Autodesk Fusion 360 part; units mm, degrees
(part 2 of 4)
sketch "Esquisse16 (2)" plane through (0, 0, 59.7937) normal (0, 0, 1) x (-1, 0, 0) in component "Left_Bottom_Holder"
  line L0 (-5.3, -152.2) -> (120.3, -152.2)
  line L1 (120.3, -152.2) -> (120.3, -145)
  line L2 (120.3, -145) -> (0, -145)
  line L3 (0, -145) -> (0, 145)
  line L4 (0, 145) -> (120.3, 145)
  line L5 (120.3, 157.8) -> (120.3, 165)
  line L6 (120.3, 165) -> (-20, 165)
  line L7 (-20, 165) -> (-20, -165)
  line L8 (-20, -165) -> (120.3, -165)
  line L9 (120.3, -165) -> (120.3, -157.8)
  line L10 (120.3, -157.8) -> (-5.3, -157.8)
  line L11 (-5.3, -157.8) -> (-5.3, -152.2)
  line L12 (0.0045, -165) -> (120.3, -165) construction
  line L13 (60.1522, -165) -> (60.15, -145) construction
  line L14 (60.1511, -155) -> (47.2609, -155.0014) construction
  line L15 (77.6517, -157.8) -> (42.6517, -157.8)
  line L16 (42.6517, -157.8) -> (42.6517, -160.3)
  line L17 (42.6517, -160.3) -> (77.6517, -160.3)
  line L18 (77.6517, -160.3) -> (77.6517, -157.8)
  line L19 (77.6505, -149.6961) -> (77.6511, -152.1961)
  line L20 (77.6511, -152.1961) -> (42.6511, -152.2039)
  line L21 (0, -145) -> (-20, -145)
  line L22 (-20, -145) -> (-20, -165)
  line L23 (-20, -165) -> (0, -165)
  line L24 (0, -165) -> (0, -145)
  line L25 (-20, 0) -> (0, 0) construction
  line L26 (-12.8, -150.3) -> (-7.2, -150.3)
  line L27 (-7.2, -150.3) -> (-7.2, 150.3)
  line L28 (-7.2, 150.3) -> (-12.8, 150.3)
  line L29 (-12.8, 150.3) -> (-12.8, -150.3)
  line L30 (-10, -165) -> (-10, -145) construction
  line L31 (0, 145) -> (-20, 145)
  line L32 (-20, 145) -> (-20, 165)
  line L33 (-20, 165) -> (0, 165)
  line L34 (0, 165) -> (0, 145)
  line L35 (-12.8, 70) -> (-12.8, -70)
  line L36 (-10, 0) -> (-10, 10) construction
  line L37 (-7.2, 70) -> (-7.2, -70)
  line L38 (0, 165) -> (120.3, 165) construction
  line L39 (60.15, 165) -> (60.15, 145) construction
  line L40 (-5.3, 157.8) -> (120.3, 157.8)
  line L41 (120.3, 152.2) -> (-5.3, 152.2)
  line L42 (-5.3, 152.2) -> (-5.3, 157.8)
  line L43 (-5.3, 157.8) -> (-5.3, 152.2)
  line L44 (-5.3, 152.2) -> (120.3, 152.2)
  line L45 (120.3, 152.2) -> (120.3, 157.8)
  line L46 (120.3, 157.8) -> (-5.3, 157.8)
  line L47 (42.65, 157.8) -> (77.65, 157.8)
  line L48 (77.65, 157.8) -> (77.65, 160.3)
  line L49 (77.65, 160.3) -> (42.65, 160.3)
  line L50 (42.65, 160.3) -> (42.65, 157.8)
  line L51 (60.15, 155) -> (66, 155) construction
  line L52 (42.65, 152.2) -> (77.65, 152.2)
  line L53 (42.65, 149.7) -> (42.65, 152.2)
  line L54 (77.65, 149.7) -> (42.65, 149.7)
  line L55 (77.65, 152.2) -> (77.65, 149.7)
  line L56 (-12.8, -90) -> (-15.3, -90)
  line L57 (-15.3, -90) -> (-15.3, -55)
  line L58 (-15.3, -55) -> (-12.8, -55)
  line L59 (-12.8, -55) -> (-12.8, -90)
  line L60 (-15.3, -90) -> (-15.3, -145) construction
  line L61 (-15.3, -55) -> (-15.3, 0) construction
  line L62 (-4.7, -90) -> (-4.7, -55)
  line L63 (-7.2, -90) -> (-4.7, -90)
  line L64 (-4.7, -55) -> (-7.2, -55)
  line L65 (-7.2, -55) -> (-7.2, -90)
  line L66 (-15.3, 90) -> (-15.3, 55)
  line L67 (-15.3, 55) -> (-12.8, 55)
  line L68 (-4.7, 90) -> (-4.7, 55)
  line L69 (-7.2, 55) -> (-7.2, 90)
  line L70 (-7.2, 90) -> (-4.7, 90)
  line L71 (-4.7, 55) -> (-7.2, 55)
  line L72 (-12.8, 90) -> (-15.3, 90)
  line L73 (-12.8, 55) -> (-12.8, 90)
  line L74 (77.6511, -152.1961) -> (42.6511, -152.2039)
  line L75 (42.6505, -149.7039) -> (77.6505, -149.6961)
  line L76 (42.6511, -152.2039) -> (42.6505, -149.7039)
  line L77 (77.6505, -149.6961) -> (77.6511, -152.1961)
  line L78 (77.6511, -152.1961) -> (42.6511, -152.2039)
  point P0 (60.1517, -160.3)
  point P1 (-10, -150.3)
  point P2 (-12.8, 0)
  point P3 (-15.3, 0)
  point P4 (60.15, 160.3)
  dimension "d128_1" = 2.5
  dimension "d129_1" = 35
  dimension "d145_1" = 5.6
  dimension "d146_1" = 300.6
  dimension "d149_1" = 2.5
  dimension "d150_1" = 35
  dimension "d236" = 2.5
  dimension "d237" = 35
  constraint coincident L8 L12.start
  constraint coincident L8.end L9.start
  constraint midpoint L12 L13.start
  constraint midpoint L2 L13.end
  constraint midpoint L13 L14.start
  constraint perpendicular L13 L14
  constraint horizontal L15
  constraint vertical L16
  constraint horizontal L17
  constraint vertical L18
  constraint coincident L10 L15.start
  constraint midpoint L17 P0
  constraint coincident L13 P0
  constraint symmetric L14 L15.start L19.end
  constraint symmetric L14 L15.end L20.end
  constraint symmetric L14 L17.end L19.start
  constraint horizontal L21
  constraint vertical L22
  constraint horizontal L23
  constraint vertical L24
  constraint coincident L7.end L8.start
  constraint coincident L2.end L3.start
  constraint midpoint L7 L25.start
  constraint coincident L25.end origin
  constraint horizontal L26
  constraint vertical L27
  constraint horizontal L28
  constraint vertical L29
  constraint midpoint L26 P1
  constraint midpoint L23 L30.start
  constraint midpoint L21 L30.end
  constraint coincident P1 L30
  constraint midpoint L29 P2
  constraint coincident L25 P2
  constraint horizontal L31
  constraint vertical L32
  constraint horizontal L33
  constraint vertical L34
  constraint coincident L6.end L7.start
  constraint coincident L3.end L4.start
  constraint vertical L35
  constraint coincident L29 L35.end
  constraint coincident L25 P3
  constraint midpoint L25 L36.start
  constraint perpendicular L25 L36
  constraint symmetric L35.end L36 L37.end
  constraint symmetric L35.start L36 L37.start
  constraint coincident L5.end L6.start
  constraint midpoint L38 L39.start
  constraint midpoint L4 L39.end
  constraint horizontal L47
  constraint vertical L48
  constraint horizontal L49
  constraint vertical L50
  constraint coincident L40 L47.start
  constraint midpoint L49 P4
  constraint coincident L39 P4
  constraint midpoint L39 L51.start
  constraint perpendicular L39 L51
  constraint symmetric L47.start L51 L52.start
  constraint symmetric L47.end L51 L52.end
  constraint symmetric L48.end L51 L54.start
  constraint symmetric L49.end L51 L53.start
  constraint horizontal L56
  constraint vertical L57
  constraint horizontal L58
  constraint vertical L59
  constraint coincident L29 L56.start
  constraint coincident L21 L60.end
  constraint perpendicular L21 L60
  constraint coincident P3 L61.end
  constraint perpendicular L25 L61
  constraint equal L60 L61
  constraint symmetric L36 L56.start L63.start
  constraint symmetric L36 L56.end L62.start
  constraint symmetric L36 L57.end L62.end
  constraint symmetric L36 L58.end L64.end
  constraint symmetric L25 L56.start L72.start
  constraint symmetric L25 L56.end L66.start
  constraint symmetric L25 L57.end L66.end
  constraint symmetric L25 L58.end L67.end
  constraint symmetric L25 L62.start L68.start
  constraint symmetric L25 L62.end L68.end
  constraint symmetric L25 L63.start L69.end
  constraint symmetric L25 L64.end L69.start
  constraint symmetric L14 L16.end L75.start
  measures "d128_1" distance of L15.end L16.end
  measures "d129_1" distance of L16.end L17.end
  measures "d145_1" distance of L26.start L26.end
  measures "d146_1" distance of L26.start L28.end
  measures "d149_1" distance of L47.start L49.end
  measures "d150_1" distance of L48.end L49.end
  measures "d236" distance of L56.start L56.end
  measures "d237" distance of L56.end L57.end
extrude "Extrusion23'" add sketch "Esquisse16 (2)" along normal blind 10 contours L0 L19 L20 L74 L75 L76 L77 L78 | L0 L20 L74 L76 L78 | L10 L15 L16 L17 L18 | L27 L37 L62 L63 L64 L65 | L27 L37 L68 L69 L70 L71 | L41 L44 L52 L53 L54 L55 | L29 L35 L56 L57 L58 L59 | L29 L35 L66 L67 L72 L73 | L40 L46 L47 L48 L49 L50 bodies 4 in component "Left_Bottom_Holder"
extrude "Extrusion28'" cut sketch "Esquisse16 (2)" against normal blind 5.3 contours L21 L26 L27 L29 | L21 L27 L29 L31 L35 L37 L59 L65 L69 L73 | L27 L28 L29 L31 bodies 4 in component "Left_Bottom_Holder"
extrude "Extrusion29'" add sketch "Esquisse16 (2)" along normal blind 30 contours L0 L7 L8 L10 L11 L21 L22 L23 L24 L26 L27 L29 | L6 L7 L27 L28 L29 L31 L32 L33 L34 L40 L41 L42 L43 L44 L46 bodies 4 in component "Left_Bottom_Holder"
sketch "Esquisse19" plane through (0, 0, 89.7937) normal (0, 0, 1) x (-1, 0, 0) in component "Left_Bottom_Holder"
  line L0 (-12.8, -150.3) -> (-12.8, -145)
  line L1 (-12.8, -145) -> (-20, -145)
  line L2 (-20, -145) -> (-20, -165)
  line L3 (-20, -165) -> (0, -165)
  line L4 (0, -165) -> (0, -157.8)
  line L5 (0, -157.8) -> (-5.3, -157.8)
  line L6 (-5.3, -157.8) -> (-5.3, -152.2)
  line L7 (-5.3, -152.2) -> (0, -152.2)
  line L8 (0, -152.2) -> (0, -145)
  line L9 (0, -145) -> (-7.2, -145)
  line L10 (-7.2, -145) -> (-7.2, -150.3)
  line L11 (-7.2, -150.3) -> (-12.8, -150.3)
  line L12 (-20, -155) -> (0, -155) construction
  line L13 (-10, -165) -> (-10, -145) construction
  circle A0 centre (-15, -155) radius 2.5
  line L14 (-10, -165) -> (-20, -165) construction
  line L15 (-15, -165) -> (-15, -145) construction
  line L16 (0, 145) -> (-20, 145) construction
  line L17 (-20, 145) -> (-20, 165) construction
  line L18 (-20, 165) -> (0, 165) construction
  line L19 (0, 165) -> (0, 145) construction
  line L20 (-10, 145) -> (-10, 165) construction
  line L21 (0, 155) -> (-20, 155) construction
  line L22 (-10, 145) -> (-20, 145) construction
  line L23 (-15, 145) -> (-15, 165) construction
  circle A1 centre (-15, 155) radius 2.5
  dimension "d155_1" = 5
  dimension "d375" = 5
  constraint midpoint L2 L12.start
  constraint perpendicular L4 L12
  constraint midpoint L3 L13.start
  constraint perpendicular L1 L13
  constraint coincident L2.end L3.start
  constraint midpoint L14 L15.start
  constraint coincident L1 L15.end
  constraint perpendicular L1 L15
  constraint midpoint A0.centre L15
  constraint horizontal L16
  constraint vertical L17
  constraint horizontal L18
  constraint vertical L19
  constraint midpoint L18 L20.end
  constraint perpendicular L18 L20
  constraint midpoint L17 L21.end
  constraint perpendicular L17 L21
  constraint perpendicular L17 L22
  constraint midpoint L22 L23.start
  constraint coincident L18 L23.end
  constraint perpendicular L18 L23
  constraint midpoint L23 A1.centre
  measures "d155_1" diameter of A0
  measures "d375" diameter of A1
extrude "Extrusion30" add sketch "Esquisse19" along normal blind 10 contours A0 | A1 bodies 4 in component "Left_Bottom_Holder"
split "Scinder1'" by plane through (-120.3, 0, 47.2937) normal (0, 1, 0) bodies 4 makes body 5 at (13.3333, 103.3333, 39.4937) in component "Left_Bottom_Holder"
move_body "Déplacer1'" bodies 4 to x (1, 0, 0) y (0, 1, 0) z (0, 0, 1) at (0, -80, 0) in component "Left_Bottom_Holder"
sketch "Esquisse21 (2)" plane through (0, -80, 0) normal (0, 1, 0) x (-1, 0, 0) in component "Left_Bottom_Holder"
  line L0 (-10, 39.7937) -> (-10, 54.4937) construction
  line L1 (-20, 49.7937) -> (-5, 49.7937) construction
  line L2 (-20, 49.7937) -> (-10, 39.7937) construction
  line L3 (-10, 49.7937) -> (-20, 39.7937) construction
  circle A0 centre (-15, 44.7937) radius 2.65
  line L4 (0, 39.4937) -> (0, 46.8437)
  line L5 (0, 46.8437) -> (-5, 46.8437)
  line L6 (-5, 46.8437) -> (-5, 52.4437)
  line L7 (-5, 52.4437) -> (0, 52.4437)
  line L8 (0, 52.4437) -> (0, 59.7937)
  line L9 (0, 59.7937) -> (-7.2, 59.7937)
  line L10 (-7.2, 59.7937) -> (-7.2, 54.4937)
  line L11 (-7.2, 54.4937) -> (-12.8, 54.4937)
  line L12 (-12.8, 54.4937) -> (-12.8, 59.7937)
  line L13 (-12.8, 59.7937) -> (-20, 59.7937)
  line L14 (-20, 59.7937) -> (-20, 39.4937)
  line L15 (-20, 39.4937) -> (0, 39.4937)
  dimension "d161_1" = 5.3
  constraint coincident L0 L3.start
  constraint coincident L1 L3.start
  constraint midpoint L3 A0.centre
  measures "d161_1" diameter of A0
extrude "Extrusion32'" cut sketch "Esquisse21 (2)" against normal blind 10.3 contours A0 bodies 4 in component "Left_Bottom_Holder"
sketch "Esquisse22 (2)" plane through (0, 0, 0) normal (0, -1, 0) x (1, 0, 0) in component "Left_Bottom_Holder"
  line L0 (10, 39.7937) -> (10, 54.4937) construction
  line L1 (20, 49.7937) -> (5, 49.7937) construction
  line L2 (20, 39.7937) -> (10, 49.7937) construction
  line L3 (10, 39.7937) -> (20, 49.7937) construction
  circle A0 centre (15, 44.7937) radius 2.5
  line L4 (0, 46.8437) -> (0, 39.4937)
  line L5 (0, 39.4937) -> (20, 39.4937)
  line L6 (20, 39.4937) -> (20, 59.7937)
  line L7 (20, 59.7937) -> (12.8, 59.7937)
  line L8 (12.8, 59.7937) -> (12.8, 54.4937)
  line L9 (12.8, 54.4937) -> (7.2, 54.4937)
  line L10 (7.2, 54.4937) -> (7.2, 59.7937)
  line L11 (7.2, 59.7937) -> (0, 59.7937)
  line L12 (0, 59.7937) -> (0, 52.4437)
  line L13 (0, 52.4437) -> (5, 52.4437)
  line L14 (5, 52.4437) -> (5, 46.8437)
  line L15 (5, 46.8437) -> (0, 46.8437)
  dimension "d164_1" = 5
  constraint coincident L1 L2.end
  constraint coincident L0 L2.end
  constraint midpoint L3 A0.centre
  measures "d164_1" diameter of A0
extrude "Extrusion33'" add sketch "Esquisse22 (2)" along normal blind 10 contours A0 bodies 5 in component "Left_Bottom_Holder"
move_body "Déplacer2'" bodies 4 to x (1, 0, 0) y (0, 1, 0) z (0, 0, 1) at (0, 80, 0) in component "Left_Bottom_Holder"
sketch "Esquisse23 (2)" plane through (0, 145, 0) normal (0, -1, 0) x (1, 0, 0) in component "Left_Bottom_Holder"
  line L0 (0, 59.7937) -> (7.2, 59.7937)
  line L1 (7.2, 59.7937) -> (7.2, 89.7937)
  line L2 (7.2, 89.7937) -> (0, 89.7937)
  line L3 (0, 89.7937) -> (0, 59.7937)
  line L4 (12.8, 59.7937) -> (20, 59.7937)
  line L5 (20, 59.7937) -> (20, 89.7937)
  line L6 (20, 89.7937) -> (12.8, 89.7937)
  line L7 (12.8, 89.7937) -> (12.8, 59.7937)
  line L8 (0, 74.7937) -> (7.2, 74.7937) construction
  line L9 (7.2, 74.7937) -> (12.8, 74.7937) construction
  line L10 (10, 74.7937) -> (10, 86.5) construction
  line L11 (7.2, 66.0437) -> (4.7, 66.0437)
  line L12 (4.7, 66.0437) -> (4.7, 83.5437)
  line L13 (4.7, 83.5437) -> (7.2, 83.5437)
  line L14 (7.2, 83.5437) -> (7.2, 66.0437)
  line L15 (15.3, 66.0437) -> (15.3, 83.5437)
  line L16 (15.3, 83.5437) -> (12.8, 83.5437)
  line L17 (12.8, 83.5437) -> (12.8, 66.0437)
  line L18 (12.8, 66.0437) -> (15.3, 66.0437)
  point P0 (4.7, 74.7937)
  dimension "d171_1" = 2.5
  dimension "d172_1" = 17.5
  constraint midpoint L3 L8.start
  constraint midpoint L1 L8.end
  constraint midpoint L7 L9.end
  constraint midpoint L9 L10.start
  constraint perpendicular L9 L10
  constraint horizontal L11
  constraint vertical L12
  constraint horizontal L13
  constraint vertical L14
  constraint coincident L1 L11.start
  constraint midpoint L12 P0
  constraint coincident L8 P0
  constraint symmetric L10 L11.start L17.end
  constraint symmetric L10 L11.end L15.start
  constraint symmetric L10 L12.end L15.end
  constraint symmetric L10 L13.end L16.end
  measures "d171_1" distance of L12.end L13.end
  measures "d172_1" distance of L11.end L12.end
extrude "Extrusion35'" add sketch "Esquisse23 (2)" along normal blind 10 contours L1 L11 L12 L13 L14 | L7 L15 L16 L17 L18 bodies 5 in component "Left_Bottom_Holder"
sketch "Esquisse24 (2)" plane through (0, -145, 0) normal (0, 1, 0) x (-1, 0, 0) in component "Left_Bottom_Holder"
  line L0 (-20, 59.7937) -> (-12.8, 59.7937)
  line L1 (-12.8, 59.7937) -> (-12.8, 89.7937)
  line L2 (-12.8, 89.7937) -> (-20, 89.7937)
  line L3 (-20, 89.7937) -> (-20, 59.7937)
  line L4 (-20, 74.7937) -> (-12.8, 74.7937) construction
  line L5 (-7.2, 59.7937) -> (0, 59.7937) construction
  line L6 (0, 59.7937) -> (0, 89.7937) construction
  line L7 (0, 89.7937) -> (-7.2, 89.7937) construction
  line L8 (-7.2, 89.7937) -> (-7.2, 59.7937) construction
  line L9 (-12.8, 74.7937) -> (-7.2, 74.7937) construction
  line L10 (-10, 74.7937) -> (-10, 87.5) construction
  line L11 (-12.8, 66.0437) -> (-15.3, 66.0437)
  line L12 (-15.3, 66.0437) -> (-15.3, 83.5437)
  line L13 (-15.3, 83.5437) -> (-12.8, 83.5437)
  line L14 (-12.8, 83.5437) -> (-12.8, 66.0437)
  line L15 (-4.7, 66.0437) -> (-4.7, 83.5437)
  line L16 (-4.7, 83.5437) -> (-7.2, 83.5437)
  line L17 (-7.2, 83.5437) -> (-7.2, 66.0437)
  line L18 (-7.2, 66.0437) -> (-4.7, 66.0437)
  point P0 (-15.3, 74.7937)
  dimension "d175_1" = 2.5
  dimension "d176_1" = 17.5
  constraint midpoint L3 L4.start
  constraint midpoint L1 L4.end
  constraint midpoint L8 L9.end
  constraint midpoint L9 L10.start
  constraint perpendicular L9 L10
  constraint horizontal L11
  constraint vertical L12
  constraint horizontal L13
  constraint vertical L14
  constraint coincident L1 L11.start
  constraint midpoint L12 P0
  constraint coincident L4 P0
  constraint symmetric L10 L11.start L17.end
  constraint symmetric L10 L11.end L15.start
  constraint symmetric L10 L12.end L15.end
  constraint symmetric L10 L13.end L16.end
  measures "d175_1" distance of L12.end L13.end
  measures "d176_1" distance of L11.end L12.end
extrude "Extrusion36'" add sketch "Esquisse24 (2)" along normal blind 10 contours L1 L11 L12 L13 L14 | L15 L16 L17 L18 bodies 4 in component "Left_Bottom_Holder"
sketch "Esquisse1 (4)" plane through (0, 0, 0) normal (1, 0, 0) x (0, 1, 0) in component "Right_Top_Holder"
  line L0 (-165, 59.7937) -> (165, 59.7937)
  line L1 (165, 59.7937) -> (165, 39.4937)
  line L2 (165, 39.4937) -> (-165, 39.4937)
  line L3 (-165, 39.4937) -> (-165, 59.7937)
  line L4 (0, 59.7937) -> (0, 39.4937) construction
  line L5 (-165, 49.6437) -> (165, 49.6437) construction
  point P0 (0, 49.6437)
  dimension "d11_2" = 330
  dimension "d12_2" = 20.3
  constraint horizontal L0
  constraint vertical L1
  constraint horizontal L2
  constraint vertical L3
  constraint midpoint L0 L4.start
  constraint midpoint L2 L4.end
  constraint midpoint L3 L5.start
  constraint midpoint L1 L5.end
  constraint midpoint L5 P0
  constraint vertical origin P0
  measures "d11_2" distance of L0.start L0.end
  measures "d12_2" distance of L0.start L2.end
extrude "Extrusion1'''" add sketch "Esquisse1 (4)" along normal blind 20 separate body makes body 6 in component "Right_Top_Holder"
sketch "Esquisse2 (3)" plane through (0, 0, 0) normal (-1, 0, 0) x (0, -1, 0) in component "Right_Top_Holder"
  line L0 (-165, 39.4937) -> (165, 39.4937)
  line L1 (165, 39.4937) -> (165, 59.7937)
  line L2 (165, 59.7937) -> (-165, 59.7937)
  line L3 (-165, 59.7937) -> (-165, 39.4937)
  line L4 (-150.3, 52.4437) -> (150.3, 52.4437)
  line L5 (150.3, 52.4437) -> (150.3, 46.8437)
  line L6 (150.3, 46.8437) -> (-150.3, 46.8437)
  line L7 (-150.3, 46.8437) -> (-150.3, 52.4437)
  line L8 (-165, 49.6437) -> (165, 49.6437) construction
  line L9 (0, 59.7937) -> (0, 39.4937) construction
  line L10 (-165, 59.7937) -> (-145, 59.7937)
  line L11 (-145, 59.7937) -> (-145, 39.4937)
  line L12 (-145, 39.4937) -> (-165, 39.4937)
  line L13 (-165, 39.4937) -> (-165, 59.7937)
  line L14 (165, 59.7937) -> (145, 59.7937)
  line L15 (145, 59.7937) -> (145, 39.4937)
  line L16 (145, 39.4937) -> (165, 39.4937)
  line L17 (165, 39.4937) -> (165, 59.7937)
  line L18 (-90, 52.4437) -> (-55, 52.4437)
  line L19 (-55, 52.4437) -> (-55, 54.9437)
  line L20 (-55, 54.9437) -> (-90, 54.9437)
  line L21 (-90, 54.9437) -> (-90, 52.4437)
  line L22 (-90, 54.9437) -> (-145, 54.9437) construction
  line L23 (-55, 54.9437) -> (0, 54.9437) construction
  line L24 (-55, 44.3437) -> (-90, 44.3437)
  line L25 (-90, 46.8437) -> (-55, 46.8437)
  line L26 (-90, 44.3437) -> (-90, 46.8437)
  line L27 (-55, 46.8437) -> (-55, 44.3437)
  line L28 (90, 54.9437) -> (90, 52.4437)
  line L29 (55, 46.8437) -> (55, 44.3437)
  line L30 (55, 52.4437) -> (55, 54.9437)
  line L31 (90, 52.4437) -> (55, 52.4437)
  line L32 (90, 46.8437) -> (55, 46.8437)
  line L33 (90, 44.3437) -> (90, 46.8437)
  line L34 (55, 44.3437) -> (90, 44.3437)
  line L35 (55, 54.9437) -> (90, 54.9437)
  point P0 (150.3, 49.6437)
  point P1 (0, 52.4437)
  point P2 (0, 53.6937)
  dimension "d16_2" = 5.6
  dimension "d17_2" = 300.6
  dimension "d109_2" = 20
  dimension "d110_2" = 20.3
  dimension "d111_2" = 20
  dimension "d112_2" = 20.3
  dimension "d238" = 2.5
  dimension "d239" = 35
  constraint horizontal L4
  constraint vertical L5
  constraint horizontal L6
  constraint vertical L7
  constraint midpoint L3 L8.start
  constraint midpoint L1 L8.end
  constraint midpoint L5 P0
  constraint coincident L8 P0
  constraint midpoint L4 P1
  constraint midpoint L2 L9.start
  constraint midpoint L0 L9.end
  constraint coincident P1 L9
  constraint coincident L9 P2
  constraint horizontal L10
  constraint vertical L11
  constraint horizontal L12
  constraint vertical L13
  constraint coincident L2.end L3.start
  constraint horizontal L14
  constraint vertical L15
  constraint horizontal L16
  constraint vertical L17
  constraint coincident L1.end L2.start
  constraint horizontal L18
  constraint vertical L19
  constraint horizontal L20
  constraint vertical L21
  constraint coincident L4 L18.start
  constraint coincident L11 L22.end
  constraint perpendicular L11 L22
  constraint coincident L9 L23.end
  constraint perpendicular L9 L23
  constraint equal L22 L23
  constraint symmetric L8 L18.start L25.start
  constraint symmetric L8 L18.end L25.end
  constraint symmetric L8 L19.end L24.start
  constraint symmetric L8 L20.end L24.end
  constraint symmetric L9 L18.start L28.end
  constraint symmetric L9 L18.end L30.start
  constraint symmetric L9 L19.end L30.end
  constraint symmetric L9 L20.end L28.start
  constraint symmetric L9 L24.start L29.end
  constraint symmetric L9 L24.end L33.start
  constraint symmetric L9 L25.start L32.start
  constraint symmetric L9 L25.end L29.start
  measures "d16_2" distance of L4 L6
  measures "d17_2" distance of L4.start L4.end
  measures "d109_2" distance of L2.end L10.end
  measures "d110_2" distance of L10.end L11.end
  measures "d111_2" distance of L1.end L14.end
  measures "d112_2" distance of L14.end L15.end
  measures "d238" distance of L18.start L20.end
  measures "d239" distance of L19.end L20.end
extrude "Extrusion2''" cut sketch "Esquisse2 (3)" against normal blind 5 contours L4 L6 L11 L15 L18 L25 L31 L32 | L4 L6 L7 L11 | L4 L5 L6 L15 bodies 6 in component "Right_Top_Holder"
extrude "Extrusion3''" add sketch "Esquisse2 (3)" along normal blind 10 contours L6 L24 L25 L26 L27 | L6 L29 L32 L33 L34 | L4 L18 L19 L20 L21 | L4 L28 L30 L31 L35 bodies 6 in component "Right_Top_Holder"
extrude "Extrusion19''" add sketch "Esquisse2 (3)" along normal blind 120.3 contours L0 L2 L3 L4 L6 L7 L10 L11 L12 L13 | L0 L1 L2 L4 L5 L6 L14 L15 L16 L17 bodies 6 in component "Right_Top_Holder"
sketch "Esquisse14 (3)" plane through (-120.3, 0, 0) normal (-1, 0, 0) x (0, -1, 0) in component "Right_Top_Holder"
  line L0 (-145, 46.8437) -> (-150.3, 46.8437)
  line L1 (-150.3, 46.8437) -> (-150.3, 52.4437)
  line L2 (-150.3, 52.4437) -> (-145, 52.4437)
  line L3 (-145, 52.4437) -> (-145, 59.7937)
  line L4 (-145, 59.7937) -> (-165, 59.7937)
  line L5 (-165, 59.7937) -> (-165, 39.4937)
  line L6 (-165, 39.4937) -> (-145, 39.4937)
  line L7 (-145, 39.4937) -> (-145, 46.8437)
  line L8 (-155, 59.7937) -> (-155, 39.4937) construction
  line L9 (-165, 49.6437) -> (-155, 49.6437) construction
  line L10 (-165, 49.6437) -> (-155, 39.4937) construction
  line L11 (-165, 39.4937) -> (-155, 49.6437) construction
  circle A0 centre (-160, 44.5687) radius 2.65
  line L12 (-157.8, 59.7937) -> (-152.2, 59.7937)
  line L13 (-152.2, 59.7937) -> (-152.2, 54.4937)
  line L14 (-152.2, 54.4937) -> (-157.8, 54.4937)
  line L15 (-157.8, 54.4937) -> (-157.8, 59.7937)
  point P0 (-155, 54.4937)
  dimension "d117_2" = 5.3
  dimension "d118_2" = 5.6
  dimension "d119_2" = 5.3
  constraint midpoint L4 L8.start
  constraint midpoint L6 L8.end
  constraint midpoint L5 L9.start
  constraint midpoint L8 L9.end
  constraint coincident L5.end L6.start
  constraint midpoint L10 A0.centre
  constraint horizontal L12
  constraint vertical L13
  constraint horizontal L14
  constraint vertical L15
  constraint coincident L4 L12.start
  constraint midpoint L14 P0
  constraint coincident L8 P0
  measures "d117_2" diameter of A0
  measures "d118_2" distance of L13.end L14.end
  measures "d119_2" distance of L12.end L13.end
extrude "Extrusion20''" cut sketch "Esquisse14 (3)" against normal blind 10.3 contours A0 bodies 6 in component "Right_Top_Holder"
extrude "Extrusion21''" cut sketch "Esquisse14 (3)" against normal up to surface (125.6 mm away) contours L4 L12 L13 L14 L15 bodies 6 in component "Right_Top_Holder"
sketch "Esquisse15 (3)" plane through (0, 145, 0) normal (0, -1, 0) x (1, 0, 0) in component "Right_Top_Holder"
  line L0 (0, 52.4437) -> (0, 59.7937)
  line L1 (0, 59.7937) -> (-120.3, 59.7937)
  line L2 (-120.3, 59.7937) -> (-120.3, 52.4437)
  line L3 (-120.3, 52.4437) -> (0, 52.4437)
  line L4 (0, 46.8437) -> (-120.3, 46.8437)
  line L5 (-120.3, 46.8437) -> (-120.3, 39.4937)
  line L6 (-120.3, 39.4937) -> (0, 39.4937)
  line L7 (-60.15, 59.7937) -> (-60.15, 52.4437) construction
  line L8 (-60.15, 52.4437) -> (-60.15, 46.8437) construction
  line L9 (-60.15, 49.6437) -> (-55, 49.6437) construction
  line L10 (-77.65, 52.4437) -> (-42.65, 52.4437)
  line L11 (-42.65, 52.4437) -> (-42.65, 54.9437)
  line L12 (-42.65, 54.9437) -> (-77.65, 54.9437)
  line L13 (-77.65, 54.9437) -> (-77.65, 52.4437)
  line L14 (-42.65, 44.3437) -> (-77.65, 44.3437)
  line L15 (-77.65, 44.3437) -> (-77.65, 46.8437)
  line L16 (-77.65, 46.8437) -> (-42.65, 46.8437)
  line L17 (-42.65, 46.8437) -> (-42.65, 44.3437)
  line L18 (0, 39.4937) -> (0, 46.8437)
  point P0 (-60.15, 54.9437)
  dimension "d124_2" = 2.5
  dimension "d125_2" = 35
  constraint midpoint L1 L7.start
  constraint midpoint L3 L7.end
  constraint midpoint L4 L8.end
  constraint midpoint L8 L9.start
  constraint perpendicular L8 L9
  constraint horizontal L10
  constraint vertical L11
  constraint horizontal L12
  constraint vertical L13
  constraint coincident L3 L10.start
  constraint midpoint L12 P0
  constraint coincident L7 P0
  constraint symmetric L9 L10.start L15.end
  constraint symmetric L9 L10.end L16.end
  constraint symmetric L9 L11.end L14.start
  constraint symmetric L9 L12.end L14.end
  measures "d124_2" distance of L10.end L11.end
  measures "d125_2" distance of L11.end L12.end
extrude "Extrusion22''" add sketch "Esquisse15 (3)" along normal blind 10 contours L3 L10 L11 L12 L13 | L4 L14 L15 L16 L17 bodies 6 in component "Right_Top_Holder"
sketch "Esquisse17 (3)" plane through (-120.3, 0, 0) normal (-1, 0, 0) x (0, -1, 0) in component "Right_Top_Holder"
  line L0 (165, 39.4937) -> (165, 59.7937)
  line L1 (165, 59.7937) -> (145, 59.7937)
  line L2 (145, 59.7937) -> (145, 52.4437)
  line L3 (145, 52.4437) -> (150.3, 52.4437)
  line L4 (150.3, 52.4437) -> (150.3, 46.8437)
  line L5 (150.3, 46.8437) -> (145, 46.8437)
  line L6 (145, 46.8437) -> (145, 39.4937)
  line L7 (145, 39.4937) -> (165, 39.4937)
  line L8 (155, 59.7937) -> (155, 39.4937) construction
  line L9 (165, 49.6437) -> (145, 49.6437) construction
  line L10 (155, 49.6437) -> (165, 39.4937) construction
  line L11 (155, 39.4937) -> (165, 49.6437) construction
  circle A0 centre (160, 44.5687) radius 2.65
  line L12 (152.2, 59.7937) -> (157.8, 59.7937)
  line L13 (157.8, 59.7937) -> (157.8, 54.4937)
  line L14 (157.8, 54.4937) -> (152.2, 54.4937)
  line L15 (152.2, 54.4937) -> (152.2, 59.7937)
  point P0 (155, 54.4937)
  dimension "d134_2" = 5.3
  dimension "d135_2" = 5.3
  dimension "d136_2" = 5.6
  constraint midpoint L1 L8.start
  constraint midpoint L7 L8.end
  constraint midpoint L0 L9.start
  constraint perpendicular L2 L9
  constraint midpoint L8 L10.start
  constraint coincident L0.start L7.end
  constraint midpoint L10 A0.centre
  constraint horizontal L12
  constraint vertical L13
  constraint horizontal L14
  constraint vertical L15
  constraint coincident L1 L12.start
  constraint midpoint L14 P0
  constraint coincident L8 P0
  measures "d134_2" diameter of A0
  measures "d135_2" distance of L12.end L13.end
  measures "d136_2" distance of L13.end L14.end
extrude "Extrusion25''" cut sketch "Esquisse17 (3)" against normal blind 10.3 contours A0 bodies 6 in component "Right_Top_Holder"
extrude "Extrusion26''" cut sketch "Esquisse17 (3)" against normal up to surface (125.6 mm away) contours L1 L12 L13 L14 L15 bodies 6 in component "Right_Top_Holder"
sketch "Esquisse18 (3)" plane through (0, -145, 0) normal (0, 1, 0) x (-1, 0, 0) in component "Right_Top_Holder"
  line L0 (0, 59.7937) -> (0, 52.4437)
  line L1 (0, 52.4437) -> (120.3, 52.4437)
  line L2 (120.3, 52.4437) -> (120.3, 59.7937)
  line L3 (120.3, 59.7937) -> (0, 59.7937)
  line L4 (0, 39.4937) -> (120.3, 39.4937) construction
  line L5 (120.3, 39.4937) -> (120.3, 46.8437) construction
  line L6 (120.3, 46.8437) -> (0, 46.8437) construction
  line L7 (60.15, 59.7937) -> (60.15, 52.4437) construction
  line L8 (60.15, 52.4437) -> (60.15, 46.8437) construction
  line L9 (60.15, 49.6437) -> (66.8882, 49.6437) construction
  line L10 (42.65, 52.4437) -> (77.65, 52.4437)
  line L11 (77.65, 52.4437) -> (77.65, 54.9437)
  line L12 (77.65, 54.9437) -> (42.65, 54.9437)
  line L13 (42.65, 54.9437) -> (42.65, 52.4437)
  line L14 (77.65, 44.3437) -> (42.65, 44.3437)
  line L15 (77.65, 46.8437) -> (77.65, 44.3437)
  line L16 (42.65, 44.3437) -> (42.65, 46.8437)
  line L17 (42.65, 46.8437) -> (77.65, 46.8437)
  line L18 (0, 46.8437) -> (0, 39.4937)
  point P0 (60.15, 54.9437)
  dimension "d141_2" = 2.5
  dimension "d142_2" = 35
  constraint midpoint L3 L7.start
  constraint midpoint L1 L7.end
  constraint midpoint L6 L8.end
  constraint midpoint L8 L9.start
  constraint perpendicular L8 L9
  constraint horizontal L10
  constraint vertical L11
  constraint horizontal L12
  constraint vertical L13
  constraint coincident L1 L10.start
  constraint midpoint L12 P0
  constraint coincident L7 P0
  constraint symmetric L9 L10.start L16.end
  constraint symmetric L9 L10.end L15.start
  constraint symmetric L9 L11.end L14.start
  constraint symmetric L9 L12.end L14.end
  measures "d141_2" distance of L10.end L11.end
  measures "d142_2" distance of L11.end L12.end
extrude "Extrusion27''" add sketch "Esquisse18 (3)" along normal blind 10 contours L1 L10 L11 L12 L13 | L14 L15 L16 L17 bodies 6 in component "Right_Top_Holder"
sketch "Esquisse16 (3)" plane through (0, 0, 59.7937) normal (0, 0, 1) x (-1, 0, 0) in component "Right_Top_Holder"
  line L0 (-5.3, -152.2) -> (120.3, -152.2)
  line L1 (120.3, -152.2) -> (120.3, -145)
  line L2 (120.3, -145) -> (0, -145)
  line L3 (0, -145) -> (0, 145)
  line L4 (0, 145) -> (120.3, 145)
  line L5 (120.3, 157.8) -> (120.3, 165)
  line L6 (120.3, 165) -> (-20, 165)
  line L7 (-20, 165) -> (-20, -165)
  line L8 (-20, -165) -> (120.3, -165)
  line L9 (120.3, -165) -> (120.3, -157.8)
  line L10 (120.3, -157.8) -> (-5.3, -157.8)
  line L11 (-5.3, -157.8) -> (-5.3, -152.2)
  line L12 (0.0094, -165) -> (120.3, -165) construction
  line L13 (60.1547, -165) -> (60.15, -145) construction
  line L14 (60.1523, -155) -> (47.2609, -155.003) construction
  line L15 (77.6628, -157.8) -> (42.6628, -157.8)
  line L16 (77.6615, -152.1918) -> (42.6615, -152.2082)
  line L17 (0, -145) -> (-20, -145)
  line L18 (-20, -145) -> (-20, -165)
  line L19 (-20, -165) -> (0, -165)
  line L20 (0, -165) -> (0, -145)
  line L21 (-20, 0) -> (0, 0) construction
  line L22 (-12.8, -150.3) -> (-7.2, -150.3)
  line L23 (-7.2, -150.3) -> (-7.2, 150.3)
  line L24 (-7.2, 150.3) -> (-12.8, 150.3)
  line L25 (-12.8, 150.3) -> (-12.8, -150.3)
  line L26 (-10, -165) -> (-10, -145) construction
  line L27 (0, 145) -> (-20, 145)
  line L28 (-20, 145) -> (-20, 165)
  line L29 (-20, 165) -> (0, 165)
  line L30 (0, 165) -> (0, 145)
  line L31 (-12.8, 70) -> (-12.8, -70)
  line L32 (-10, 0) -> (-10, 10) construction
  line L33 (-7.2, 70) -> (-7.2, -70)
  line L34 (0, 165) -> (120.3, 165) construction
  line L35 (60.15, 165) -> (60.15, 145) construction
  line L36 (-5.3, 157.8) -> (120.3, 157.8)
  line L37 (120.3, 152.2) -> (-5.3, 152.2)
  line L38 (-5.3, 152.2) -> (-5.3, 157.8)
  line L39 (-5.3, 157.8) -> (-5.3, 152.2)
  line L40 (-5.3, 152.2) -> (120.3, 152.2)
  line L41 (120.3, 152.2) -> (120.3, 157.8)
  line L42 (120.3, 157.8) -> (-5.3, 157.8)
  line L43 (42.65, 157.8) -> (77.65, 157.8)
  line L44 (60.15, 155) -> (66, 155) construction
  line L45 (42.65, 152.2) -> (77.65, 152.2)
  line L46 (-12.8, -55) -> (-12.8, -90)
  line L47 (-7.2, -55) -> (-7.2, -90)
  line L48 (-7.2, 55) -> (-7.2, 90)
  line L49 (-12.8, 55) -> (-12.8, 90)
  point P0 (60.1536, -160.15)
  point P1 (-10, -150.3)
  point P2 (-12.8, 0)
  point P3 (-15.15, 0)
  point P4 (60.15, 160.15)
  dimension "d145_2" = 5.6
  dimension "d146_2" = 300.6
  constraint coincident L8 L12.start
  constraint coincident L8.end L9.start
  constraint midpoint L12 L13.start
  constraint midpoint L2 L13.end
  constraint midpoint L13 L14.start
  constraint perpendicular L13 L14
  constraint horizontal L15
  constraint coincident L10 L15.start
  constraint coincident L13 P0
  constraint symmetric L14 L15.start L16.start
  constraint symmetric L14 L15.end L16.end
  constraint horizontal L17
  constraint vertical L18
  constraint horizontal L19
  constraint vertical L20
  constraint coincident L7.end L8.start
  constraint coincident L2.end L3.start
  constraint midpoint L7 L21.start
  constraint coincident L21.end origin
  constraint horizontal L22
  constraint vertical L23
  constraint horizontal L24
  constraint vertical L25
  constraint midpoint L22 P1
  constraint midpoint L19 L26.start
  constraint midpoint L17 L26.end
  constraint coincident P1 L26
  constraint midpoint L25 P2
  constraint coincident L21 P2
  constraint horizontal L27
  constraint vertical L28
  constraint horizontal L29
  constraint vertical L30
  constraint coincident L6.end L7.start
  constraint coincident L3.end L4.start
  constraint vertical L31
  constraint coincident L25 L31.end
  constraint coincident L21 P3
  constraint midpoint L21 L32.start
  constraint perpendicular L21 L32
  constraint symmetric L31.end L32 L33.end
  constraint symmetric L31.start L32 L33.start
  constraint coincident L5.end L6.start
  constraint midpoint L34 L35.start
  constraint midpoint L4 L35.end
  constraint horizontal L43
  constraint coincident L36 L43.start
  constraint coincident L35 P4
  constraint midpoint L35 L44.start
  constraint perpendicular L35 L44
  constraint symmetric L43.start L44 L45.start
  constraint symmetric L43.end L44 L45.end
  constraint vertical L46
  constraint coincident L25 L46.end
  constraint symmetric L32 L46.end L47.end
  constraint symmetric L32 L46.start L47.start
  constraint symmetric L21 L46.end L49.end
  constraint symmetric L21 L46.start L49.start
  constraint symmetric L21 L47.end L48.end
  constraint symmetric L21 L47.start L48.start
  measures "d145_2" distance of L22.start L22.end
  measures "d146_2" distance of L22.start L24.end
extrude "Extrusion28''" cut sketch "Esquisse16 (3)" against normal blind 5.3 contours L17 L22 L23 L25 | L17 L23 L25 L27 L31 L33 L46 L47 L48 L49 | L23 L24 L25 L27 bodies 6 in component "Right_Top_Holder"
extrude "Extrusion29''" add sketch "Esquisse16 (3)" along normal blind 30 contours L0 L7 L8 L10 L11 L17 L18 L19 L20 L22 L23 L25 | L6 L7 L23 L24 L25 L27 L28 L29 L30 L36 L37 L38 L39 L40 L42 bodies 6 in component "Right_Top_Holder"
sketch "Esquisse19 (2)" plane through (0, 0, 89.7937) normal (0, 0, 1) x (-1, 0, 0) in component "Right_Top_Holder"
  line L0 (-12.8, -150.3) -> (-12.8, -145)
  line L1 (-12.8, -145) -> (-20, -145)
  line L2 (-20, -145) -> (-20, -165)
  line L3 (-20, -165) -> (0, -165)
  line L4 (0, -165) -> (0, -157.8)
  line L5 (0, -157.8) -> (-5.3, -157.8)
  line L6 (-5.3, -157.8) -> (-5.3, -152.2)
  line L7 (-5.3, -152.2) -> (0, -152.2)
  line L8 (0, -152.2) -> (0, -145)
  line L9 (0, -145) -> (-7.2, -145)
  line L10 (-7.2, -145) -> (-7.2, -150.3)
  line L11 (-7.2, -150.3) -> (-12.8, -150.3)
  line L12 (-20, -155) -> (0, -155) construction
  line L13 (-10, -165) -> (-10, -145) construction
  line L14 (-10, -165) -> (-20, -165) construction
  line L15 (-15, -165) -> (-15, -145) construction
  circle A0 centre (-15, -155) radius 2.65
  line L16 (0, 145) -> (-20, 145) construction
  line L17 (-20, 145) -> (-10, 145) construction
  line L18 (-10, 165) -> (-10, 145) construction
  line L19 (-10, 155) -> (-20, 155) construction
  line L20 (-15, 145) -> (-15, 165) construction
  circle A1 centre (-15, 155) radius 2.65
  dimension "d360" = 5.3
  dimension "d361" = 5.3
  constraint midpoint L2 L12.start
  constraint perpendicular L4 L12
  constraint midpoint L3 L13.start
  constraint perpendicular L1 L13
  constraint coincident L2.end L3.start
  constraint midpoint L14 L15.start
  constraint coincident L1 L15.end
  constraint perpendicular L1 L15
  constraint midpoint L15 A0.centre
  constraint horizontal L16
  constraint midpoint L16 L17.end
  constraint perpendicular L16 L18
  constraint midpoint L18 L19.start
  constraint perpendicular L18 L19
  constraint midpoint L17 L20.start
  constraint perpendicular L19 L20
  constraint midpoint L19 A1.centre
  measures "d360" diameter of A0
  measures "d361" diameter of A1
extrude "Extrusion30'" cut sketch "Esquisse19 (2)" against normal blind 10.3 contours A0 | A1 bodies 6 in component "Right_Top_Holder"
split "Scinder1''" by plane through (-120.3, 0, 47.2937) normal (0, 1, 0) bodies 6 makes body 7 at (13.3333, 103.3333, 39.4937) in component "Right_Top_Holder"
move_body "Déplacer1''" bodies 6 to x (1, 0, 0) y (0, 1, 0) z (0, 0, 1) at (0, -80, 0) in component "Right_Top_Holder"
sketch "Esquisse21 (3)" plane through (0, -80, 0) normal (0, 1, 0) x (-1, 0, 0) in component "Right_Top_Holder"
  line L0 (-10, 39.7937) -> (-10, 54.4937) construction
  line L1 (-20, 49.7937) -> (-5, 49.7937) construction
  line L2 (-20, 49.7937) -> (-10, 39.7937) construction
  line L3 (-10, 49.7937) -> (-20, 39.7937) construction
  circle A0 centre (-15, 44.7937) radius 2.65
  line L4 (0, 39.4937) -> (0, 46.8437)
  line L5 (0, 46.8437) -> (-5, 46.8437)
  line L6 (-5, 46.8437) -> (-5, 52.4437)
  line L7 (-5, 52.4437) -> (0, 52.4437)
  line L8 (0, 52.4437) -> (0, 59.7937)
  line L9 (0, 59.7937) -> (-7.2, 59.7937)
  line L10 (-7.2, 59.7937) -> (-7.2, 54.4937)
  line L11 (-7.2, 54.4937) -> (-12.8, 54.4937)
  line L12 (-12.8, 54.4937) -> (-12.8, 59.7937)
  line L13 (-12.8, 59.7937) -> (-20, 59.7937)
  line L14 (-20, 59.7937) -> (-20, 39.4937)
  line L15 (-20, 39.4937) -> (0, 39.4937)
  dimension "d161_2" = 5.3
  constraint coincident L0 L3.start
  constraint coincident L1 L3.start
  constraint midpoint L3 A0.centre
  measures "d161_2" diameter of A0
extrude "Extrusion32''" cut sketch "Esquisse21 (3)" against normal blind 10.3 contours A0 bodies 6 in component "Right_Top_Holder"
sketch "Esquisse22 (3)" plane through (0, 0, 0) normal (0, -1, 0) x (1, 0, 0) in component "Right_Top_Holder"
  line L0 (10, 39.7937) -> (10, 54.4937) construction
  line L1 (20, 49.7937) -> (5, 49.7937) construction
  line L2 (20, 39.7937) -> (10, 49.7937) construction
  line L3 (10, 39.7937) -> (20, 49.7937) construction
  circle A0 centre (15, 44.7937) radius 2.5
  line L4 (0, 46.8437) -> (0, 39.4937)
  line L5 (0, 39.4937) -> (20, 39.4937)
  line L6 (20, 39.4937) -> (20, 59.7937)
  line L7 (20, 59.7937) -> (12.8, 59.7937)
  line L8 (12.8, 59.7937) -> (12.8, 54.4937)
  line L9 (12.8, 54.4937) -> (7.2, 54.4937)
  line L10 (7.2, 54.4937) -> (7.2, 59.7937)
  line L11 (7.2, 59.7937) -> (0, 59.7937)
  line L12 (0, 59.7937) -> (0, 52.4437)
  line L13 (0, 52.4437) -> (5, 52.4437)
  line L14 (5, 52.4437) -> (5, 46.8437)
  line L15 (5, 46.8437) -> (0, 46.8437)
  dimension "d164_2" = 5
  constraint coincident L1 L2.end
  constraint coincident L0 L2.end
  constraint midpoint L3 A0.centre
  measures "d164_2" diameter of A0
extrude "Extrusion33''" add sketch "Esquisse22 (3)" along normal blind 10 contours A0 bodies 7 in component "Right_Top_Holder"
move_body "Déplacer2''" bodies 6 to x (1, 0, 0) y (0, 1, 0) z (0, 0, 1) at (0, 80, 0) in component "Right_Top_Holder"
sketch "Esquisse1 (5)" plane through (0, 0, 0) normal (1, 0, 0) x (0, 1, 0) in component "Left_Top_Holder"
  line L0 (-165, 59.7937) -> (165, 59.7937)
  line L1 (165, 59.7937) -> (165, 39.4937)
  line L2 (165, 39.4937) -> (-165, 39.4937)
  line L3 (-165, 39.4937) -> (-165, 59.7937)
  line L4 (0, 59.7937) -> (0, 39.4937) construction
  line L5 (-165, 49.6437) -> (165, 49.6437) construction
  point P0 (0, 49.6437)
  dimension "d11_1_1" = 330
  dimension "d12_1_1" = 20.3
  constraint horizontal L0
  constraint vertical L1
  constraint horizontal L2
  constraint vertical L3
  constraint midpoint L0 L4.start
  constraint midpoint L2 L4.end
  constraint midpoint L3 L5.start
  constraint midpoint L1 L5.end
  constraint midpoint L5 P0
  constraint vertical origin P0
  measures "d11_1_1" distance of L0.start L0.end
  measures "d12_1_1" distance of L0.start L2.end
extrude "Extrusion1''''" add sketch "Esquisse1 (5)" along normal blind 20 separate body makes body 8 in component "Left_Top_Holder"
sketch "Esquisse2 (4)" plane through (0, 0, 0) normal (-1, 0, 0) x (0, -1, 0) in component "Left_Top_Holder"
  line L0 (-165, 39.4937) -> (165, 39.4937)
  line L1 (165, 39.4937) -> (165, 59.7937)
  line L2 (165, 59.7937) -> (-165, 59.7937)
  line L3 (-165, 59.7937) -> (-165, 39.4937)
  line L4 (-150.3, 52.4437) -> (150.3, 52.4437)
  line L5 (150.3, 52.4437) -> (150.3, 46.8437)
  line L6 (150.3, 46.8437) -> (-150.3, 46.8437)
  line L7 (-150.3, 46.8437) -> (-150.3, 52.4437)
  line L8 (-165, 49.6437) -> (165, 49.6437) construction
  line L9 (0, 59.7937) -> (0, 39.4937) construction
  line L10 (-165, 59.7937) -> (-145, 59.7937)
  line L11 (-145, 59.7937) -> (-145, 39.4937)
  line L12 (-145, 39.4937) -> (-165, 39.4937)
  line L13 (-165, 39.4937) -> (-165, 59.7937)
  line L14 (165, 59.7937) -> (145, 59.7937)
  line L15 (145, 59.7937) -> (145, 39.4937)
  line L16 (145, 39.4937) -> (165, 39.4937)
  line L17 (165, 39.4937) -> (165, 59.7937)
  line L18 (-90, 52.4437) -> (-55, 52.4437)
  line L19 (-90, 46.8437) -> (-55, 46.8437)
  line L20 (90, 52.4437) -> (55, 52.4437)
  point P0 (150.3, 49.6437)
  point P1 (0, 52.4437)
  point P2 (0, 53.6937)
  dimension "d16_1_1" = 5.6
  dimension "d17_1_1" = 300.6
  dimension "d109_1_1" = 20
  dimension "d110_1_1" = 20.3
  dimension "d111_1_1" = 20
  dimension "d112_1_1" = 20.3
  constraint horizontal L4
  constraint vertical L5
  constraint horizontal L6
  constraint vertical L7
  constraint midpoint L3 L8.start
  constraint midpoint L1 L8.end
  constraint midpoint L5 P0
  constraint coincident L8 P0
  constraint midpoint L4 P1
  constraint midpoint L2 L9.start
  constraint midpoint L0 L9.end
  constraint coincident P1 L9
  constraint coincident L9 P2
  constraint horizontal L10
  constraint vertical L11
  constraint horizontal L12
  constraint vertical L13
  constraint coincident L2.end L3.start
  constraint horizontal L14
  constraint vertical L15
  constraint horizontal L16
  constraint vertical L17
  constraint coincident L1.end L2.start
  constraint horizontal L18
  constraint coincident L4 L18.start
  constraint symmetric L8 L18.start L19.start
  constraint symmetric L8 L18.end L19.end
  constraint symmetric L9 L18.start L20.start
  constraint symmetric L9 L18.end L20.end
  measures "d16_1_1" distance of L4 L6
  measures "d17_1_1" distance of L4.start L4.end
  measures "d109_1_1" distance of L2.end L10.end
  measures "d110_1_1" distance of L10.end L11.end
  measures "d111_1_1" distance of L1.end L14.end
  measures "d112_1_1" distance of L14.end L15.end
extrude "Extrusion2'''" cut sketch "Esquisse2 (4)" against normal blind 5 contours L4 L6 L11 L15 L18 L19 L20 | L4 L6 L7 L11 | L4 L5 L6 L15 bodies 8 in component "Left_Top_Holder"
extrude "Extrusion19'''" add sketch "Esquisse2 (4)" along normal blind 120.3 contours L0 L2 L3 L4 L6 L7 L10 L11 L12 L13 | L0 L1 L2 L4 L5 L6 L14 L15 L16 L17 bodies 8 in component "Left_Top_Holder"
sketch "Esquisse14 (4)" plane through (-120.3, 0, 0) normal (-1, 0, 0) x (0, -1, 0) in component "Left_Top_Holder"
  line L0 (-145, 46.8437) -> (-150.3, 46.8437)
  line L1 (-150.3, 46.8437) -> (-150.3, 52.4437)
  line L2 (-150.3, 52.4437) -> (-145, 52.4437)
  line L3 (-145, 52.4437) -> (-145, 59.7937)
  line L4 (-145, 59.7937) -> (-165, 59.7937)
  line L5 (-165, 59.7937) -> (-165, 39.4937)
  line L6 (-165, 39.4937) -> (-145, 39.4937)
  line L7 (-145, 39.4937) -> (-145, 46.8437)
  line L8 (-155, 59.7937) -> (-155, 39.4937) construction
  line L9 (-165, 49.6437) -> (-155, 49.6437) construction
  line L10 (-165, 49.6437) -> (-155, 39.4937) construction
  line L11 (-165, 39.4937) -> (-155, 49.6437) construction
  circle A0 centre (-160, 44.5687) radius 2.5
  line L12 (-157.8, 59.7937) -> (-152.2, 59.7937)
  line L13 (-152.2, 59.7937) -> (-152.2, 54.4937)
  line L14 (-152.2, 54.4937) -> (-157.8, 54.4937)
  line L15 (-157.8, 54.4937) -> (-157.8, 59.7937)
  point P0 (-155, 54.4937)
  dimension "d117_1_1" = 5
  dimension "d118_1_1" = 5.6
  dimension "d119_1_1" = 5.3
  constraint midpoint L4 L8.start
  constraint midpoint L6 L8.end
  constraint midpoint L5 L9.start
  constraint midpoint L8 L9.end
  constraint coincident L5.end L6.start
  constraint midpoint L10 A0.centre
  constraint horizontal L12
  constraint vertical L13
  constraint horizontal L14
  constraint vertical L15
  constraint coincident L4 L12.start
  constraint midpoint L14 P0
  constraint coincident L8 P0
  measures "d117_1_1" diameter of A0
  measures "d118_1_1" distance of L13.end L14.end
  measures "d119_1_1" distance of L12.end L13.end
extrude "Extrusion20'''" add sketch "Esquisse14 (4)" along normal blind 10 contours A0 bodies 8 in component "Left_Top_Holder"
extrude "Extrusion21'''" cut sketch "Esquisse14 (4)" against normal up to surface (125.6 mm away) contours L4 L12 L13 L14 L15 bodies 8 in component "Left_Top_Holder"
sketch "Esquisse17 (4)" plane through (-120.3, 0, 0) normal (-1, 0, 0) x (0, -1, 0) in component "Left_Top_Holder"
  line L0 (165, 39.4937) -> (165, 59.7937)
  line L1 (165, 59.7937) -> (145, 59.7937)
  line L2 (145, 59.7937) -> (145, 52.4437)
  line L3 (145, 52.4437) -> (150.3, 52.4437)
  line L4 (150.3, 52.4437) -> (150.3, 46.8437)
  line L5 (150.3, 46.8437) -> (145, 46.8437)
  line L6 (145, 46.8437) -> (145, 39.4937)
  line L7 (145, 39.4937) -> (165, 39.4937)
  line L8 (155, 59.7937) -> (155, 39.4937) construction
  line L9 (165, 49.6437) -> (145, 49.6437) construction
  line L10 (155, 49.6437) -> (165, 39.4937) construction
  line L11 (155, 39.4937) -> (165, 49.6437) construction
  circle A0 centre (160, 44.5687) radius 2.5
  line L12 (152.2, 59.7937) -> (157.8, 59.7937)
  line L13 (157.8, 59.7937) -> (157.8, 54.4937)
  line L14 (157.8, 54.4937) -> (152.2, 54.4937)
  line L15 (152.2, 54.4937) -> (152.2, 59.7937)
  point P0 (155, 54.4937)
  dimension "d134_1_1" = 5
  dimension "d135_1_1" = 5.3
  dimension "d136_1_1" = 5.6
  constraint midpoint L1 L8.start
  constraint midpoint L7 L8.end
  constraint midpoint L0 L9.start
  constraint perpendicular L2 L9
  constraint midpoint L8 L10.start
  constraint coincident L0.start L7.end
  constraint midpoint L10 A0.centre
  constraint horizontal L12
  constraint vertical L13
  constraint horizontal L14
  constraint vertical L15
  constraint coincident L1 L12.start
  constraint midpoint L14 P0
  constraint coincident L8 P0
  measures "d134_1_1" diameter of A0
  measures "d135_1_1" distance of L12.end L13.end
  measures "d136_1_1" distance of L13.end L14.end
extrude "Extrusion25'''" add sketch "Esquisse17 (4)" along normal blind 10 contours A0 bodies 8 in component "Left_Top_Holder"
extrude "Extrusion26'''" cut sketch "Esquisse17 (4)" against normal up to surface (125.6 mm away) contours L1 L12 L13 L14 L15 bodies 8 in component "Left_Top_Holder"